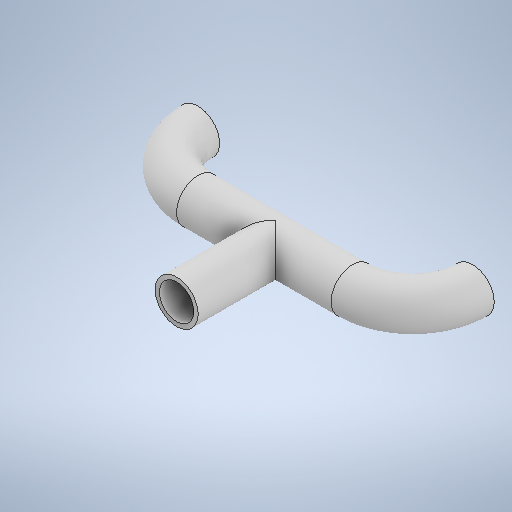
# Autodesk Inventor part: 25
Saved by Autodesk Inventor 2025.1 (Build 291241000, 241)
## iProperties
Created: 2024-09-13
Part Number: 25
Material: Generisch
Document SubType Name: Modeling
Designer: ffogue
Density: 1 g/cm^3
Appearance: Vorgabe
Author: ffogue
Autodesk Inventor part; units mm, degrees
ref_plane "YZ Plane" through (0, 0, 0) normal (1, 0, 0) x (0, 1, 0)
ref_plane "XY Plane" through (0, 0, 0) normal (0, 0, 1) x (1, 0, 0)
sketch "Sketch1" plane through (0, 0, 0) normal (0, 1, 0) x (-1, 0, 0)
  circle A0 centre (0, 0) radius 2.5
  circle A1 centre (0, 0) radius 2
  dimension "d0" = 5
  dimension "d1" = 4
  constraints: 2 centre point, 2 coincident
  measures "d0" diameter of A0
  measures "d1" diameter of A1
sketch "Sketch2" plane through (0, 0, 0) normal (0, 0, 1) x (1, 0, 0)
  line L0 (0, 0) -> (0, 0)
  line L1 (7, -7) -> (25, -7)
  line L2 (32, 0) -> (32, 0)
  arc A0 (0, 0) -> (7, -7) centre (7, 0) ccw
  arc A1 (25, -7) -> (32, 0) centre (25, 0) ccw
  point P0 (0, -7)
  point P1 (32, -7)
  dimension "d3" = 32
  dimension "d4" = 7
  dimension "d5" = 7
  constraints: 6 end point, 4 point on circle, 4 point on line, 4 tangent, 2 centre point, 1 coincident, 1 horizontal alignment, 1 parallel, 1 perpendicular, 1 vertical, 1 vertical alignment
  measures "d3" distance of point (0, -7) point (32, -7)
  measures "d4" radius of A0
  measures "d5" radius of A1
sweep "Sweep1" add profiles "Sketch1" path "Sketch2"
ref_plane "Work Plane1" through (0, -18.5, 0) normal (0, 1, 0) x (-1, 0, 0)
sketch "Sketch3" plane through (0, -18.5, 0) normal (0, 1, 0) x (-1, 0, 0)
  circle A0 centre (-16, 0) radius 2.5
  circle A1 centre (0, 0) radius 2.5 projected
  circle A2 centre (-16, 0) radius 2
  dimension "d9" = 5
  dimension "d10" = 16
  dimension "d11" = 4
  constraints: 2 centre point, 1 coincident, 1 horizontal alignment
  measures "d9" diameter of A0
  measures "d10" distance of A1.centre A0.centre
  measures "d11" diameter of A2
extrude "Extrusion1" add sketch "Sketch3" along normal up to surface contours A0
body "Solid1"
